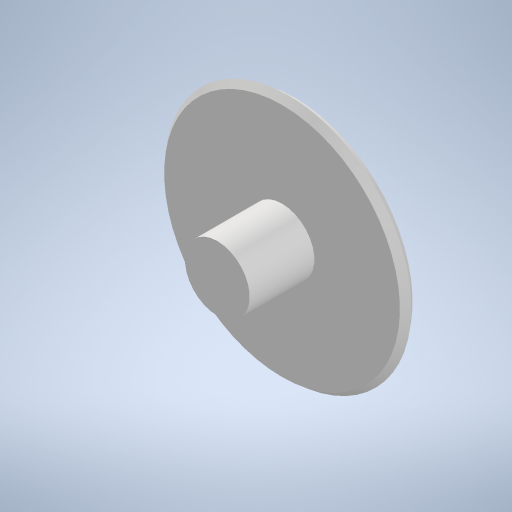
# Autodesk Inventor part: Ventosa
Saved by Autodesk Inventor 2023.1 (Build 271208000, 208)
## iProperties
Created: 2022-11-04
Part Number: Ventosa
Material: Generic
Document SubType Name: Modeling
Designer: Daniel Peña
Density: 1 g/cm^3
Appearance: Default
Author: Daniel Peña
Autodesk Inventor part; units mm, degrees
ref_plane "YZ Plane" through (0, 0, 0) normal (1, 0, 0) x (0, 1, 0)
ref_plane "XZ Plane" through (0, 0, 0) normal (0, 1, 0) x (-1, 0, 0)
ref_plane "XY Plane" through (0, 0, 0) normal (0, 0, 1) x (1, 0, 0)
sketch "Sketch2" plane through (0, 0, 0) normal (1, 0, 0) x (0, 1, 0)
  line L0 (12.5, 0) -> (22.75, 0)
  line L1 (22.75, 2.45) -> (6.25, 2.45)
  line L2 (0, 14.95) -> (0, 0)
  line L3 (22.75, 2.45) -> (22.75, 0) construction
  line L4 (22.75, 1.225) -> (23.75, 1.225) construction
  line L5 (22.75, 2.45) -> (23.75, 1.225)
  line L6 (22.75, 0) -> (23.75, 1.225)
  line L7 (6.25, 2.45) -> (6.25, 14.95)
  line L8 (6.25, 14.95) -> (0, 14.95)
  line L9 (22.6076, 0.3) -> (12.5, 0.3)
  line L10 (0, 2.15) -> (22.6076, 2.15)
  line L11 (22.6076, 2.15) -> (23.3627, 1.225)
  line L12 (23.3627, 1.225) -> (22.6076, 0.3)
  line L13 (12.5, 0) -> (12.5, 0.3)
  point P0 (0, 0.3)
  dimension "d0" = 45.5
  dimension "d1" = 2.45
  dimension "d2" = 1
  dimension "d4" = 12.5
  dimension "d6" = 12.5
  dimension "d7" = 0.3
  constraints: 28 end point, 4 vertical, 3 horizontal, 2 parallel, 2 point on line, 1 midpoint, 1 other
  measures "d0" diameter of L0.end L2
  measures "d1" distance between parallel lines of L1 L0
  measures "d2" distance of L4.start L4.end
  measures "d4" diameter of L7 L2
  measures "d6" distance of L1.end L7.end
  measures "d7" distance between parallel lines of L0 L9
revolve "Revolution1" add sketch "Sketch2" angle 360 about axis through (0, 0, 14.95) along (0, 0, -1)
body "Solid1"
